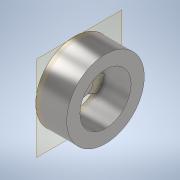
# Autodesk Inventor part: Reaction_wheel_dr - Copy (3.3)
Saved by Autodesk Inventor 2021.1 (Build 251245010, 245A)
## iProperties
Created: 2022-01-30
Part Number: Reaction_wheel_dr - Copy (3.3)
Material: Steel, Carbon
Document SubType Name: Modeling
Designer: D3rrick
Density: 7.85 g/cm^3
Appearance: Semi-Polished
Mass: 80.5142 g
Surface Area: 67.4268 cm^2
Volume: 10.2566 cm^3
Author: D3rrick
Autodesk Inventor part; units mm, degrees
ref_plane "YZ Plane" through (0, 0, 0) normal (1, 0, 0) x (0, 1, 0)
ref_plane "XZ Plane" through (0, 0, 0) normal (0, 1, 0) x (-1, 0, 0)
ref_plane "XY Plane" through (0, 0, 0) normal (0, 0, 1) x (1, 0, 0)
sketch "Sketch1" plane through (0, 0, 0) normal (1, 0, 0) x (0, 1, 0)
  circle A0 centre (0, 0) radius 6
  dimension "hubouter" = 12
  constraints: 1 centre point, 1 coincident
  measures "hubouter" diameter of A0
extrude "Extrusion1" add sketch "Sketch1" along normal blind 6
sketch "Sketch2" plane through (0, 0, 0) normal (-1, 0, 0) x (0, 0, 1)
  circle A0 centre (0, 0) radius 1.5
  dimension "hole" = 3
  constraints: 1 centre point, 1 coincident
  measures "hole" diameter of A0
hole "Hole1" at (0, 0, 0) direction (1, 0, 0) diameter 5.5 end through all
sketch "Sketch3" plane through (0, 0, 0) normal (-1, 0, 0) x (0, 0, 1)
  circle A0 centre (0, 0) radius 16.5
  circle A1 centre (0, 0) radius 25
  circle A2 centre (0, 0) radius 6 projected
  line L0 (6, 0) -> (26, 0)
  line L1 (16.1025, -3.6) -> (4.8, -3.6)
  line L2 (16.1025, 3.6) -> (4.8, 3.6)
  arc A3 (4.8, -3.6) -> (4.8, 3.6) centre (0, 0) ccw
  dimension "innerdiam" = 33
  dimension "outerdiam" = 50
  constraints: 6 end point, 5 point on circle, 2 centre point, 2 coincident, 2 symmetric about line, 1 horizontal, 1 parallel, 3 other
  measures "outerdiam" diameter of A1
extrude "Extrusion2" add sketch "Sketch3" against normal blind 20
sketch "Sketch5" plane through (0, 0, 0) normal (1, 0, 0) x (0, 1, 0)
  circle A0 centre (0, 0) radius 6 construction
  line L0 (0, 6) -> (22.3607, 6)
  circle A1 centre (0, 0) radius 2.75 projected
  line L1 (0, -6) -> (23.0083, -2.5724)
  line L2 (23.0083, -2.5724) -> (22.7003, -2.6183)
  arc A2 (0, -6) -> (0, 6) centre (0, 0) ccw
  arc A3 (23.0083, -2.5724) -> (22.3607, 6) centre (0, 0) ccw
  point P0 (1.7489, -5.7395)
  constraints: 7 end point, 4 point on circle, 2 centre point, 2 coincident, 2 horizontal, 1 point on line, 1 vertical alignment, 2 other
extrude "Extrusion4" add sketch "Sketch5" along normal blind 3 contours L0 A3 L1 A2
pattern_circular "Circular Pattern2" count 3 over 360 about axis through (-10, 0, 0) along (1, 0, 0) of "Extrusion4"
ref_plane "Work Plane4" through (3, 16.1022, -3.6012) normal (1, 0, 0) x (0, 1, 0)
body "Solid1"
